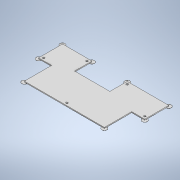
# Autodesk Inventor part: TopPlate
Saved by Autodesk Inventor 2020 (Build 240168000, 168)
## iProperties
Created: 2024-02-29
Part Number: TopPlate
Material: Generic
Document SubType Name: Modeling
Designer: smz3rm
Density: 1 g/cm^3
Appearance: Default
Author: smz3rm
Autodesk Inventor part; units mm, degrees
ref_plane "YZ Plane" through (0, 0, 0) normal (1, 0, 0) x (0, 1, 0)
ref_plane "XZ Plane" through (0, 0, 0) normal (0, 1, 0) x (-1, 0, 0)
ref_plane "XY Plane" through (0, 0, 0) normal (0, 0, 1) x (1, 0, 0)
sketch "Sketch1" plane through (0, 0, 0) normal (0, 1, 0) x (-1, 0, 0)
  line L0 (-12.7, 8) -> (8, 8) projected
  line L1 (8, 8) -> (-12.7, 8)
  line L2 (8, 8) -> (8, -29.85) projected
  line L3 (8, 8) -> (8, -29.85)
  line L4 (-38.6, -29.85) -> (-38.6, -21.85) projected
  line L5 (8, -29.85) -> (-38.6, -29.85)
  line L6 (-38.6, -2.35) -> (-38.6, -21.85) projected
  line L7 (-38.6, -29.85) -> (-38.6, -2.35)
  line L8 (-94.4, -2.35) -> (-38.6, -2.35) projected
  line L9 (-38.6, -2.35) -> (-94.4, -2.35)
  line L10 (-94.4, -21.85) -> (-94.4, -29.85) projected
  line L11 (-94.4, -2.35) -> (-94.4, -29.85)
  line L12 (-94.4, -29.85) -> (-160, -29.85) projected
  line L13 (-94.4, -29.85) -> (-160, -29.85)
  line L14 (-160, -29.85) -> (-160, 8) projected
  line L15 (-160, -29.85) -> (-160, 8)
  line L16 (-139.3, 8) -> (-139.3, 51.15) projected
  line L17 (-160, 8) -> (-139.3, 8)
  line L18 (-139.3, 8) -> (-139.3, 51.15)
  line L19 (-139.3, 51.15) -> (-12.7, 51.15) projected
  line L20 (-139.3, 51.15) -> (-12.7, 51.15)
  line L21 (-12.7, 51.15) -> (-12.7, 8) projected
  line L22 (-12.7, 51.15) -> (-12.7, 8)
  circle A0 centre (-34.6, -25.85) radius 1.875 projected
  circle A1 centre (-34.6, -25.85) radius 1.55
  circle A2 centre (4, 4) radius 1.55
  circle A3 centre (-76, 47.15) radius 1.55
  circle A4 centre (-156, 4) radius 1.55
  circle A5 centre (-98.4, -25.85) radius 1.55
  point P0 (0, 0)
  dimension "d2" = 3.1
  constraints: 24 end point, 9 coincident, 8 perpendicular, 5 centre point, 4 equal radius, 2 collinear
  measures "d2" diameter of A1
extrude "Extrusion1" add sketch "Sketch1" along normal blind 1.5 contours L0 L2 L5 L4 L6 L8 L11 L10 L12 L14 L17 L16 L19 L21 | A0
sketch "Sketch2" plane through (0, 0, 0) normal (0, -1, 0) x (1, 0, 0)
  line L0 (12.7, 8) -> (12.7, 51.15) projected
  circle A0 centre (12.7, 51.15) radius 4
  line L1 (12.7, 51.15) -> (139.3, 51.15) projected
  circle A1 centre (139.3, 51.15) radius 4
  line L2 (160, 8) -> (160, -29.85) projected
  circle A2 centre (160, 8) radius 4
  circle A3 centre (160, -29.85) radius 4
  circle A4 centre (94.4, -29.85) radius 4
  circle A5 centre (38.4923, -29.85) radius 4
  line L3 (38.6, -29.85) -> (-8, -29.85) projected
  circle A6 centre (-8, -29.85) radius 4
  circle A7 centre (-8, 8) radius 4
  point P0 (0, 0)
  dimension "d7" = 8
  dimension "d8" = 8
  dimension "d9" = 8
  dimension "d10" = 8
  dimension "d11" = 8
  dimension "d12" = 8
  dimension "d13" = 8
  dimension "d14" = 8
  constraints: 8 centre point, 1 coincident
  measures "d7" diameter of A0
  measures "d8" diameter of A1
  measures "d9" diameter of A2
  measures "d10" diameter of A3
  measures "d11" diameter of A4
  measures "d12" diameter of A5
  measures "d13" diameter of A6
  measures "d14" diameter of A7
extrude "Extrusion2" add sketch "Sketch2" against normal blind 0.2
body "Solid1"
